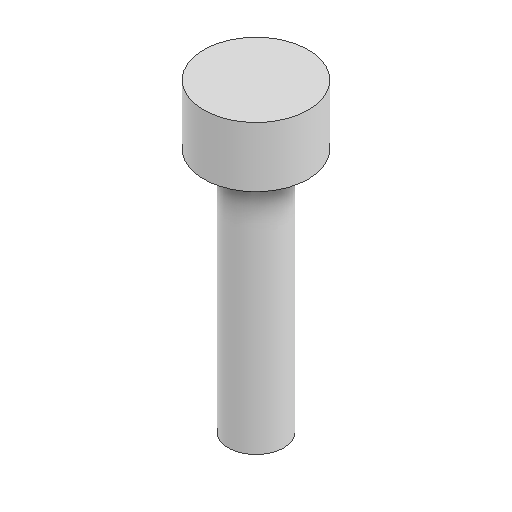
# Autodesk Inventor part: Screw BIG 3
Saved by Autodesk Inventor 2025 (Build 290162010, 162A)
## iProperties
Created: 2024-12-04
Part Number: Screw BIG 3
Material: Generic
Document SubType Name: Modeling
Designer: ALEXANDERNICHOLS
Density: 1 g/cm^3
Appearance: Default
Author: ALEXANDERNICHOLS
Autodesk Inventor part; units mm, degrees
ref_plane "YZ Plane" through (0, 0, 0) normal (1, 0, 0) x (0, 1, 0)
ref_plane "XZ Plane" through (0, 0, 0) normal (0, 1, 0) x (-1, 0, 0)
ref_plane "XY Plane" through (0, 0, 0) normal (0, 0, 1) x (1, 0, 0)
sketch "Sketch1" plane through (0, 0, 0) normal (0, 0, 1) x (1, 0, 0)
  line L0 (0, 0) -> (1.778, 0)
  line L1 (1.778, 0) -> (1.778, 15.7988)
  line L2 (1.778, 15.7988) -> (3.3655, 15.7988)
  line L3 (3.3655, 15.7988) -> (3.3655, 19.6596)
  line L4 (3.3655, 19.6596) -> (0, 19.6596)
  line L5 (0, 19.6596) -> (0, 0)
  dimension "d1" = 6.731
  dimension "d2" = 3.556
  dimension "d3" = 3.8608
  dimension "d4" = 15.7988
  constraints: 12 end point, 4 perpendicular, 1 horizontal, 1 vertical
  measures "d1" diameter of L3 L5
  measures "d2" diameter of L1 L5
  measures "d3" distance of L2.end L3.end
  measures "d4" distance of L0.end L1.end
revolve "Revolution1" add sketch "Sketch1" angle 360 about axis through (0, 19.6596, 0) along (0, -1, 0)
body "Solid1"
